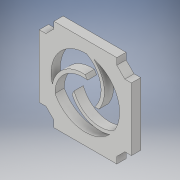
# Autodesk Inventor part: 20_Cube_Insert_Objective_Holder_v3
Saved by Autodesk Inventor 2019 (Build 230136000, 136)
## iProperties
Created: 2019-07-01
Part Number: 20_Cube_Insert_Objective_Holder_v3
Material: Generic
Document SubType Name: Modeling
Designer: diederichbenedict
Density: 1 g/cm^3
Appearance: Default
Author: diederichbenedict
Autodesk Inventor part; units mm, degrees
ref_plane "YZ Plane" through (0, 0, 0) normal (1, 0, 0) x (0, 1, 0)
ref_plane "Work Plane1" through (0, 0, 10) normal (0, 0, 1) x (1, 0, 0)
sketch "Sketch1" plane through (0, 0, 10) normal (0, 0, 1) x (1, 0, 0)
  line L0 (-4.0299, -0.3538) -> (-2.2322, 1.4439) construction
  arc A0 (-1.4439, 2.2322) -> (-2.2322, 1.4439) centre (-0.9299, 0.9299) ccw construction
  line L1 (-1.4439, 2.2322) -> (0.3538, 4.0299) construction
  line L2 (-37.8299, 42.2137) -> (-37.8299, 45.8299) construction
  line L3 (-37.8299, 45.8299) -> (-4.0299, 45.8299) construction
  line L4 (-4.0299, 45.8299) -> (-4.0299, 42.2137) construction
  line L5 (-4.0299, 4.0299) -> (0.3538, 4.0299) projected
  line L6 (-20.9299, 58.9723) -> (17.1124, 20.9299) construction
  line L7 (17.1124, 20.9299) -> (-20.9299, -17.1124) construction
  line L8 (-20.9299, -17.1124) -> (-58.9723, 20.9299) construction
  line L9 (-58.9723, 20.9299) -> (-20.9299, 58.9723) construction
  line L10 (-20.9299, 58.9723) -> (-20.9299, -17.1124) construction
  line L11 (17.1124, 20.9299) -> (-58.9723, 20.9299) construction
  line L12 (-20.9299, 58.9723) -> (32.8701, 58.9723) construction
  line L13 (-43.4299, 43.4299) -> (1.5701, 43.4299) construction
  line L14 (1.5701, 43.4299) -> (1.5701, -1.5701) construction
  line L15 (1.5701, -1.5701) -> (-43.4299, -1.5701) construction
  line L16 (-43.4299, -1.5701) -> (-43.4299, 43.4299) construction
  line L17 (-43.4299, 43.4299) -> (1.5701, -1.5701) construction
  line L18 (1.5701, 43.4299) -> (-43.4299, -1.5701) construction
  line L19 (-43.4299, 5.3876) -> (-43.4299, 36.4723)
  line L20 (-43.4299, 36.4723) -> (-36.4723, 43.4299)
  line L21 (-36.4723, 43.4299) -> (-5.3876, 43.4299)
  line L22 (-5.3876, 43.4299) -> (1.5701, 36.4723)
  line L23 (1.5701, 36.4723) -> (1.5701, 5.3876)
  line L24 (1.5701, 5.3876) -> (-5.3876, -1.5701)
  line L25 (-5.3876, -1.5701) -> (-36.4723, -1.5701)
  line L26 (-36.4723, -1.5701) -> (-43.4299, 5.3876)
  line L27 (-4.0299, 42.2137) -> (-37.8299, 42.2137) projected
  line L28 (-4.0299, -0.3538) -> (-4.0299, 4.0299) projected
  circle A1 centre (-20.9299, 20.9299) radius 13.3985
  circle A2 centre (-20.9299, 20.9299) radius 15.4895
  point P0 (-37.8299, 4.0299)
  dimension "d18" = 53.8
  dimension "d19" = 45
  dimension "d20" = 53.8
  dimension "d21" = 45
  dimension "d22" = 45
  dimension "d30" = 26.797
  dimension "d36" = 30.979
  constraints: 42 end point, 15 point on line, 4 parallel, 3 midpoint, 3 perpendicular, 2 centre point, 2 coincident, 2 horizontal, 1 equal length
  measures "d18" distance of L6.start L6.end
  measures "d19" angle of L6 L12
  measures "d20" distance of L6.end L7.end
  measures "d21" distance of L14.end L15.end
  measures "d22" distance of L13.end L14.end
  measures "d30" diameter of A1
  measures "d36" diameter of A2
extrude "Extrusion1" add sketch "Sketch1" along normal blind 5 contours L28 L24 L25 L26 L19 L20 L27 L22 L23 L5 | L5 L24 L28 | L27 L20 L21 L22 | A1 | A2
ref_plane "Work Plane2" through (-40.9959, 0.8639, 22.2359) normal (0, 0, 1) x (1, 0, 0)
sketch "Sketch3" plane through (0, 0, 10) normal (0, 0, -1) x (-1, 0, 0)
  line L0 (37.8299, -0.4701) -> (37.8299, 4.0299) construction
  line L1 (4.0299, 4.0299) -> (4.0299, -0.4701) construction
  line L2 (37.8299, -0.4701) -> (37.8299, 1.1886) construction
  line L3 (4.0299, -3.9701) -> (4.0299, -0.3538) construction
  line L4 (45.8299, 4.0299) -> (42.2137, 4.0299) construction
  line L5 (-0.3538, 4.0299) -> (-3.9701, 4.0299) construction
  line L6 (-3.9701, 37.8299) -> (-0.3538, 37.8299) construction
  line L7 (4.0299, 42.2137) -> (4.0299, 45.8299) construction
  line L8 (37.8299, 45.8299) -> (37.8299, 42.2137) construction
  line L9 (42.2137, 37.8299) -> (45.8299, 37.8299) construction
  line L10 (37.8299, 37.7299) -> (45.8299, 37.7299)
  line L11 (45.8299, 37.7299) -> (45.8299, 4.1299)
  line L12 (45.8299, 4.1299) -> (37.8299, 4.1299)
  line L13 (37.8299, 4.1299) -> (37.8299, 37.7299)
  line L14 (37.7299, 4.0299) -> (4.1299, 4.0299)
  line L15 (4.1299, 4.0299) -> (4.1299, -3.9701)
  line L16 (4.1299, -3.9701) -> (37.7299, -3.9701)
  line L17 (37.7299, -3.9701) -> (37.7299, 4.0299)
  line L18 (4.0299, 4.1299) -> (-3.9701, 4.1299)
  line L19 (-3.9701, 4.1299) -> (-3.9701, 37.7299)
  line L20 (-3.9701, 37.7299) -> (4.0299, 37.7299)
  line L21 (4.0299, 37.7299) -> (4.0299, 4.1299)
  line L22 (4.1299, 37.8299) -> (37.7299, 37.8299)
  line L23 (37.7299, 37.8299) -> (37.7299, 45.8299)
  line L24 (37.7299, 45.8299) -> (4.1299, 45.8299)
  line L25 (4.1299, 45.8299) -> (4.1299, 37.8299)
  point P0 (0, 0)
  dimension "d23" = 0.1
  dimension "d24" = 0.1
  dimension "d25" = 0.1
  dimension "d26" = 0.1
  dimension "d27" = 0.1
  constraints: 32 end point, 8 parallel, 4 horizontal, 4 perpendicular, 3 point on line
  measures "d23" distance between parallel lines of L8 L23
  measures "d24" distance between parallel lines of L7 L25
  measures "d25" distance between parallel lines of L6 L20
  measures "d26" distance between parallel lines of L5 L18
  measures "d27" distance between parallel lines of L1 L15
extrude "Extrusion3" add sketch "Sketch3" against normal up to surface (5 mm away)
sketch "Sketch6" plane through (0, 0, 15) normal (0, 0, 1) x (1, 0, 0)
  circle A0 centre (-20.9299, 20.9299) radius 18.5
  circle A1 centre (-20.9299, 20.9299) radius 13.3985
  line L0 (-45.8299, 4.1299) -> (-45.8299, 37.7299) projected
  line L1 (-4.1299, -3.9701) -> (-37.7299, -3.9701) projected
  line L2 (-37.7299, 45.8299) -> (-4.1299, 45.8299) projected
  point P0 (0, 0)
  point P1 (-45.8299, 20.9299)
  point P2 (-20.9299, -3.9701)
  point P3 (-20.9299, 45.8299)
  dimension "d37" = 26.797
  dimension "d38" = 37
  constraints: 3 midpoint, 2 centre point, 2 vertical alignment, 1 coincident, 1 horizontal alignment
  measures "d37" diameter of A1
  measures "d38" diameter of A0
extrude "Extrusion5" cut sketch "Sketch6" against normal blind 12 contours A0 | A1
sketch "Sketch7" plane through (0, 0, 15) normal (0, 0, 1) x (1, 0, 0)
  arc A0 (-7.3514, 4.1907) -> (-4.1915, 7.0829) centre (-15.9478, 16.7551) ccw
  arc A1 (-7.3514, 4.1907) -> (-4.1915, 7.0829) centre (-15.9478, 16.7551) ccw
  circle A2 centre (-20.9299, 20.9299) radius 18.5 construction
  circle A3 centre (-20.9299, 20.9299) radius 6.5 construction
  arc A4 (-15.9478, 16.7551) -> (-20.1559, 39.4137) centre (-27.3968, 26.3489) ccw
  arc A5 (-13.6076, 16.8625) -> (-16.2405, 38.8257) centre (-27.3968, 26.3489) ccw
  arc A6 (-16.2405, 38.8257) -> (-20.1559, 39.4137) centre (-20.9299, 20.9299) ccw
  line L0 (-15.9478, 16.7551) -> (-13.6076, 16.8625)
  point P0 (0, 0)
  point P1 (-25.3654, 35.7708)
  point P2 (-14.2, -44.8454)
  point P3 (-13.5804, 16.4347)
  point P4 (-13.5804, 8.5029)
  dimension "d79" = 13
  dimension "d83" = 1.8
  constraints: 12 point on circle, 6 centre point, 2 coincident, 2 end point, 1 tangent, 4 other
  measures "d79" diameter of A3
  measures "d83" radial gap between concentric circles of A4 A5
extrude "Extrusion6" add sketch "Sketch7" against normal up to surface (5 mm away)
pattern_circular "Circular Pattern1" count 3 over 360 about axis through (-20.9299, 20.9299, 15) along (0, 0, -1) of "Extrusion6"
sketch "Skizze11" plane through (0, 0, 15) normal (0, 0, 1) x (1, 0, 0)
  arc A0 (-5.3095, 11.0177) -> (-16.2405, 38.8257) centre (-20.9299, 20.9299) ccw construction
  arc A1 (-27.0364, 18.7027) -> (-5.3095, 11.0177) centre (-13.0035, 23.8209) ccw construction
  line L0 (-28.1135, 16.6223) -> (-27.0364, 18.7027) construction
  arc A2 (-28.1135, 16.6223) -> (-7.7764, 7.9209) centre (-13.0035, 23.8209) ccw construction
  arc A3 (-37.3244, 12.3584) -> (-7.7764, 7.9209) centre (-20.9299, 20.9299) ccw construction
  arc A4 (-19.8055, 27.3319) -> (-37.3244, 12.3584) centre (-22.3895, 12.6199) ccw construction
  line L1 (-21.0686, 29.3049) -> (-19.8055, 27.3319) construction
  arc A5 (-21.0686, 29.3049) -> (-38.7728, 16.0432) centre (-22.3895, 12.6199) ccw construction
  arc A6 (-20.1559, 39.4137) -> (-38.7728, 16.0432) centre (-20.9299, 20.9299) ccw construction
  arc A7 (-15.9478, 16.7551) -> (-20.1559, 39.4137) centre (-27.3968, 26.3489) ccw construction
  line L2 (-13.6076, 16.8625) -> (-15.9478, 16.7551) construction
  arc A8 (-13.6076, 16.8625) -> (-16.2405, 38.8257) centre (-27.3968, 26.3489) ccw construction
  line L3 (3.9701, 4.1299) -> (0.3124, 4.1299) projected
  line L4 (3.9701, 37.7299) -> (3.9701, 4.1299) construction
  line L5 (0.3124, 37.7299) -> (3.9701, 37.7299) projected
  line L6 (0.3124, 37.7299) -> (-4.1299, 42.1723) projected
  line L7 (-4.1299, 45.8299) -> (-4.1299, 42.1723) projected
  line L8 (-37.7299, 45.8299) -> (-4.1299, 45.8299) construction
  line L9 (-37.7299, 42.1723) -> (-37.7299, 45.8299) projected
  line L10 (-37.7299, 42.1723) -> (-42.1723, 37.7299) projected
  line L11 (-45.8299, 37.7299) -> (-42.1723, 37.7299) projected
  line L12 (-45.8299, 4.1299) -> (-45.8299, 37.7299) construction
  line L13 (-42.1723, 4.1299) -> (-45.8299, 4.1299) projected
  line L14 (-42.1723, 4.1299) -> (-37.7299, -0.3124) projected
  line L15 (-37.7299, -3.9701) -> (-37.7299, -0.3124) projected
  line L16 (-4.1299, -3.9701) -> (-37.7299, -3.9701) construction
  line L17 (-4.1299, -0.3124) -> (-4.1299, -3.9701) projected
  line L18 (-4.1299, -0.3124) -> (0.3124, 4.1299) projected
  line L19 (-3.9299, 46.0299) -> (-3.9299, 42.2551)
  line L20 (-3.9299, 42.2551) -> (0.3953, 37.9299)
  line L21 (0.3953, 37.9299) -> (4.1701, 37.9299)
  line L22 (4.1701, 37.9299) -> (4.1701, 3.9299) construction
  line L23 (4.1701, 3.9299) -> (0.3953, 3.9299)
  line L24 (0.3953, 3.9299) -> (-3.9299, -0.3953)
  line L25 (-3.9299, -0.3953) -> (-3.9299, -4.1701)
  line L26 (-3.9299, -4.1701) -> (-37.9299, -4.1701) construction
  line L27 (-37.9299, -4.1701) -> (-37.9299, -0.3953)
  line L28 (-37.9299, -0.3953) -> (-42.2551, 3.9299)
  line L29 (-42.2551, 3.9299) -> (-46.0299, 3.9299)
  line L30 (-46.0299, 3.9299) -> (-46.0299, 37.9299) construction
  line L31 (-46.0299, 37.9299) -> (-42.2551, 37.9299)
  line L32 (-42.2551, 37.9299) -> (-37.9299, 42.2551)
  line L33 (-37.9299, 42.2551) -> (-37.9299, 46.0299)
  line L34 (-37.9299, 46.0299) -> (-3.9299, 46.0299) construction
  line L35 (-45.8299, 37.7299) -> (-45.8299, 37.9299)
  line L36 (-37.7299, 45.8299) -> (-37.9299, 45.8299)
  line L37 (-4.1299, 45.8299) -> (-3.9299, 45.8299)
  line L38 (3.9701, 37.7299) -> (3.9701, 37.9299)
  line L39 (3.9701, 37.7299) -> (3.9701, 4.1299) projected
  line L40 (3.9701, 4.1299) -> (3.9701, 3.9299)
  line L41 (-4.1299, -3.9701) -> (-3.9299, -3.9701)
  line L42 (-37.7299, -3.9701) -> (-37.9299, -3.9701)
  line L43 (-45.8299, 4.1299) -> (-45.8299, 3.9299)
  point P0 (0, 0)
  dimension "d84" = 0.2
  constraints: 48 end point, 12 point on line, 4 perpendicular, 15 other
  measures "d84" distance between parallel lines of L8 L34
extrude "IM_offset" add sketch "Skizze11" against normal up to surface (5 mm away)
body "Solid1"
